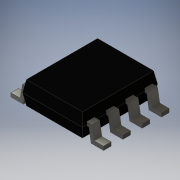
# Autodesk Inventor part: SO-8
Saved by Autodesk Inventor 2016 (Build 200138000, 138)
## iProperties
Created: 2017-03-04
Part Number: SO-8
Material: Generic
Document SubType Name: Modeling
Designer: jfixelle
Density: 1 g/cm^3
Appearance: Smooth - Black
Author: jfixelle
Autodesk Inventor part; units mm, degrees
ref_plane "YZ Plane" through (0, 0, 0) normal (1, 0, 0) x (0, 1, 0)
ref_plane "XZ Plane" through (0, 0, 0) normal (0, 1, 0) x (-1, 0, 0)
sketch "Sketch1" plane through (0, 0, 0) normal (0, 1, 0) x (-1, 0, 0)
  line L0 (1.975, 2.475) -> (-1.975, 2.475)
  line L1 (-1.975, 2.475) -> (-1.975, -2.475)
  line L2 (-1.975, -2.475) -> (1.975, -2.475)
  line L3 (1.975, -2.475) -> (1.975, 2.475)
  point P0 (0, 0)
  dimension "d0" = 3.95
  dimension "d1" = 1.975
  dimension "d2" = 4.95
  dimension "d3" = 2.475
  constraints: 8 end point, 2 parallel, 1 horizontal, 1 perpendicular
  measures "d0" distance of L1.end L2.end
  measures "d1" distance from line of point (0, 0) L3
  measures "d2" distance of L2.end L0.start
  measures "d3" distance from line of point (0, 0) L2
extrude "Extrusion1" add sketch "Sketch1" along normal blind 1.5
chamfer "Chamfer1" distance 0.75 angle 10 1 edges at (0, 1.5, 2.475) measured on face at (-0.6583, 0.5, 2.475)
chamfer "Chamfer2" distance 0.75 angle 10 1 edges at (1.975, 1.5, -0.0661) measured on face at (1.975, 1, -0.8691)
chamfer "Chamfer3" distance 0.75 angle 10 1 edges at (-0.0661, 1.5, -2.475) measured on face at (-0.6583, 0.75, -2.475)
chamfer "Chamfer4" distance 0.75 angle 10 1 edges at (-1.975, 1.5, 0) measured on face at (-1.975, 0.5, 0.825)
chamfer "Chamfer5" distance 0.75 angle 10 1 edges at (-1.975, 0, 0) measured on face at (-1.975, 0.25, -0.825)
chamfer "Chamfer6" distance 0.75 angle 10 1 edges at (0.0661, 0, -2.475) measured on face at (-0.6143, 0.5, -2.475)
chamfer "Chamfer7" distance 0.75 angle 10 1 edges at (1.975, 0, 0.0661) measured on face at (1.975, 0.5, -0.781)
chamfer "Chamfer8" distance 0.75 angle 10 1 edges at (0, 0, 2.475) measured on face at (0.6143, 0.4999, 2.475)
ref_plane "Work Plane1" through (0, 0, 0.635) normal (0, 0, 1) x (1, 0, 0)
sketch "Sketch2" plane through (0, 0, 0.635) normal (0, 0, 1) x (1, 0, 0)
  line L0 (1.8485, 0.9035) -> (1.8485, 0.6535)
  line L1 (1.8485, 0.6535) -> (2.0795, 0.6535)
  line L2 (2.0795, 0.6535) -> (2.23, -0.2)
  line L3 (2.23, -0.2) -> (3.05, -0.2)
  line L4 (3.05, -0.2) -> (3.05, 0.05)
  line L5 (3.05, 0.05) -> (2.4398, 0.05)
  line L6 (2.4398, 0.05) -> (2.2893, 0.9035)
  line L7 (1.8485, 0.9035) -> (2.2893, 0.9035)
  line L8 (-1.8428, 0) -> (1.8428, 0) projected
  line L9 (0, 0) -> (0, -0.508)
  dimension "d31" = 0.2
  dimension "d32" = 0.82
  dimension "d33" = 3.05
  dimension "d34" = 0.25
  dimension "d35" = 0.25
  dimension "d36" = 0.25
  dimension "d37" = 80
  constraints: 18 end point, 3 perpendicular, 1 horizontal, 1 parallel, 1 vertical
  measures "d31" distance between parallel lines of L8 L3
  measures "d32" distance of L2.end L3.end
  measures "d33" distance between parallel lines of L4 L9
  measures "d34" distance between parallel lines of L3 L5
  measures "d35" distance between parallel lines of L1 L7
  measures "d36" distance between parallel lines of L2 L6
  measures "d37" angle of L6 L5
extrude "Extrusion2" add sketch "Sketch2" along normal mid plane 0.5
pattern_linear "Rectangular Pattern1" count 4 spacing 1.27 along (0, 0, -1) of "Extrusion2" first direction both ways yes
mirror "Mirror1" about plane through (0, 0, 0) normal (1, 0, 0) of "Extrusion2", "Rectangular Pattern1"
body "Solid1"
